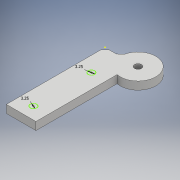
# Autodesk Inventor part: revHinge1
Saved by Autodesk Inventor 2018.2 (Build 222227000, 227)
## iProperties
Created: 2018-03-30
Part Number: revHinge1
Material: Generic
Document SubType Name: Modeling
Designer: mzhang
Density: 1 g/cm^3
Appearance: Default
Author: mzhang
Autodesk Inventor part; units mm, degrees
ref_plane "YZ Plane" through (0, 0, 0) normal (1, 0, 0) x (0, 1, 0)
ref_plane "XZ Plane" through (0, 0, 0) normal (0, 1, 0) x (-1, 0, 0)
ref_plane "XY Plane" through (0, 0, 0) normal (0, 0, 1) x (1, 0, 0)
sketch "Sketch1" plane through (0, 0, 0) normal (0, 0, 1) x (1, 0, 0)
  line L0 (0, 0) -> (15, 0)
  line L1 (15, 0) -> (15, -50)
  line L2 (15, -50) -> (0, -50)
  line L3 (0, -50) -> (0, 0)
  circle A0 centre (16.75, 0) radius 1.75
  circle A1 centre (16.75, 0) radius 9.0322
  dimension "d12" = 3.5
  dimension "d0" = 15
  dimension "d1" = 50
  constraints: 8 end point, 2 parallel, 1 centre point, 1 coincident, 1 horizontal, 1 horizontal alignment, 1 perpendicular, 2 other
  measures "d0" distance of L1.end L2.end
  measures "d1" distance of L0.end L1.end
extrude "Extrusion1" add sketch "Sketch1" along normal blind 4
chamfer "Chamfer1" distance 2 angle 45 1 edges at (7.7178, 0, 2)
chamfer "Chamfer2" distance 2 angle 45 1 edges at (0, 0, 2)
sketch "Sketch2" plane through (0, 0, 4) normal (0, 0, 1) x (1, 0, 0)
  circle A0 centre (7.5, -43.8644) radius 1.625
  circle A1 centre (7.5, -14.4752) radius 1.625
  point P0 (0, 0)
  dimension "d10" = 3.25
  dimension "d11" = 3.25
  constraints: 2 centre point
  measures "d10" diameter of A0
  measures "d11" diameter of A1
body "Solid1"
